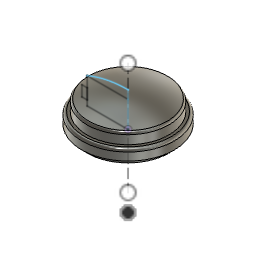
Druckknopf v5 (Autodesk Fusion 360 design; units mm, degrees)
Autodesk Fusion 360 part; units mm, degrees
sketch "Skizze1" plane through (0, 0, 0) normal (0, 1, 0) x (1, 0, 0)
  line L0 (-7.8, -5) -> (0, -5)
  line L1 (0, -5) -> (0, 0)
  line L2 (0, 0) -> (-7.8, 0)
  line L3 (-7.8, 0) -> (-7.8, -5)
  line L4 (0, -10.9451) -> (0, 10.4416) construction
  arc A0 (-7.8, -5) -> (0, -6.5584) centre (0, 13.7403) ccw
  line L5 (0, -6.5584) -> (0, -5)
  line L6 (-7.8, -1) -> (-8.8, -1)
  line L7 (-8.8, -1) -> (-8.8, -3)
  line L8 (-8.8, -3) -> (-7.8, -3)
  line L9 (-7.8, -3) -> (-7.8, -1)
  dimension "d2" = 7.8
  dimension "d20" = 5
  dimension "d21" = 17
  dimension "d29" = 1
  dimension "d30" = 2
  dimension "d31" = 1
  constraint horizontal L0
  constraint horizontal L2
  constraint vertical L3
  constraint perpendicular L2 L4
  constraint coincident L2.start L1
  constraint coincident L1.end L4
  constraint coincident L4 A0.centre
  constraint perpendicular L0 L5
  constraint coincident L1.end L2
  constraint horizontal L6
  constraint vertical L7
  constraint horizontal L8
  constraint vertical L9
  constraint coincident L3 L6.start
  measures "d2" distance of L1.end L3
  measures "d20" distance of L0 L2
  measures "d21" distance of L4.end A0.end
  measures "d29" distance of L3 L7
  measures "d30" distance of L6 L8
  measures "d31" distance of L2 L6
revolve "Drehen3" add sketch "Skizze1" angle 360 about axis through (0, 0, 10.9451) along (0, 0, -1)
fillet "Abrundung1" radius 0.5 1 edges at (-7.2722, 2.8206, 5)
fillet "Abrundung3" radius 0.5 1 edges at (-8.2045, 3.1822, 3)
fillet "Abrundung4" radius 0.5 1 edges at (-7.2722, 2.8206, 1)
